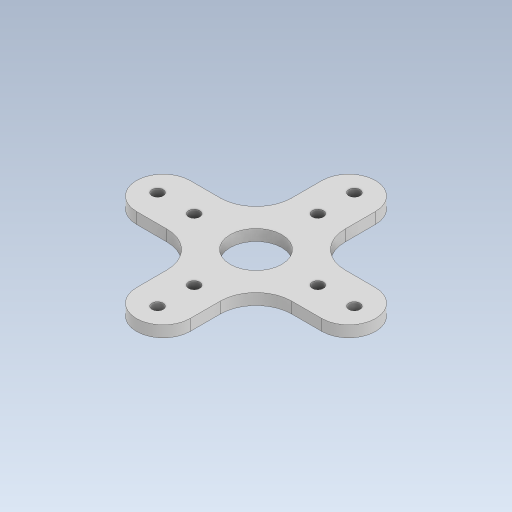
# Autodesk Inventor part: DriveMotorPlate
Saved by Autodesk Inventor 2023 (Build 270158000, 158)
## iProperties
Created: 2023-03-28
Part Number: DriveMotorPlate
Material: Generic
Document SubType Name: Modeling
Designer: Dave
Density: 1 g/cm^3
Appearance: Default
Author: Dave
Autodesk Inventor part; units mm, degrees
ref_plane "YZ Plane" through (0, 0, 0) normal (1, 0, 0) x (0, 1, 0)
ref_plane "XZ Plane" through (0, 0, 0) normal (0, 1, 0) x (-1, 0, 0)
ref_plane "XY Plane" through (0, 0, 0) normal (0, 0, 1) x (1, 0, 0)
sketch "Sketch1" plane through (0, 0, 0) normal (0, 1, 0) x (-1, 0, 0)
  line L0 (-9.525, -33) -> (-9.525, -22.225)
  line L1 (-9.525, 22.225) -> (-9.525, 33)
  line L2 (33, 9.525) -> (22.225, 9.525)
  line L3 (-22.225, 9.525) -> (-33, 9.525)
  line L4 (9.525, 33) -> (9.525, 22.225)
  line L5 (9.525, -22.225) -> (9.525, -33)
  line L6 (-33, -9.525) -> (-22.225, -9.525)
  line L7 (22.225, -9.525) -> (33, -9.525)
  line L8 (77.6073, 0) -> (-79.7857, 0) projected
  line L9 (0, -77.9019) -> (0, 71.2895) projected
  circle A0 centre (-35, 0) radius 2
  circle A1 centre (-22, 0) radius 2
  circle A2 centre (0, -22) radius 2
  circle A3 centre (0, -35) radius 2
  circle A4 centre (22, 0) radius 2
  circle A5 centre (35, 0) radius 2
  circle A6 centre (0, 22) radius 2
  circle A7 centre (0, 35) radius 2
  circle A8 centre (0, 0) radius 9.185
  line L10 (-57.3009, 49.9764) -> (55.1226, 49.9764) construction
  line L11 (55.1226, 49.9764) -> (55.1226, -56.5889) construction
  line L12 (55.1226, -56.5889) -> (-57.3009, -56.5889) construction
  line L13 (-57.3009, -56.5889) -> (-57.3009, 49.9764) construction
  arc A9 (9.525, 33) -> (0, 42.525) centre (0, 33) ccw
  arc A10 (0, 42.525) -> (-9.525, 33) centre (0, 33) ccw
  arc A11 (42.525, 0) -> (33, 9.525) centre (33, 0) ccw
  arc A12 (33, -9.525) -> (42.525, 0) centre (33, 0) ccw
  arc A13 (0, -42.525) -> (9.525, -33) centre (0, -33) ccw
  arc A14 (-9.525, -33) -> (0, -42.525) centre (0, -33) ccw
  arc A15 (-42.525, 0) -> (-33, -9.525) centre (-33, 0) ccw
  arc A16 (-33, 9.525) -> (-42.525, 0) centre (-33, 0) ccw
  arc A17 (9.525, 22.225) -> (22.225, 9.525) centre (22.225, 22.225) ccw
  arc A18 (22.225, -9.525) -> (9.525, -22.225) centre (22.225, -22.225) ccw
  arc A19 (-9.525, -22.225) -> (-22.225, -9.525) centre (-22.225, -22.225) ccw
  arc A20 (-22.225, 9.525) -> (-9.525, 22.225) centre (-22.225, 22.225) ccw
  point P0 (0, 42.525)
  point P1 (42.525, 0)
  point P2 (0, -42.525)
  point P3 (-42.525, 0)
  point P4 (42.525, 0)
  point P5 (0, 42.525)
  point P6 (-42.525, 0)
  dimension "d2" = 360
  dimension "d4" = 4
  dimension "d5" = 22
  dimension "d6" = 35
  dimension "d7" = 18.37
  dimension "d39" = 9.525
  dimension "d41" = 9.525
  dimension "d46" = 12.7
  constraints: 24 point on circle, 20 centre point, 16 end point, 16 tangent, 10 equal radius, 8 parallel, 7 point on line, 4 horizontal, 3 perpendicular, 3 vertical, 1 coincident, 1 vertical alignment, 45 other
  measures "d4" diameter of A0
  measures "d5" distance from line of A1.centre L9
  measures "d6" distance from line of L9 A0.centre
  measures "d7" diameter of A8
  measures "d39" radius of A9
  measures "d41" radius of A14
  measures "d46" radius of A17
extrude "Extrusion1" add sketch "Sketch1" along normal blind 4 contours L0 A19 L6 A15 L8 A0 A1 A8 L9 A2 A3 A14 | L9 A3 A2 A8 L8 A4 A5 A12 L7 A18 L5 A13 | A16 L3 A20 L1 A10 L9 A7 A6 A8 L8 A1 A0 | L8 A5 A4 A8 L9 A6 A7 A9 L4 A17 L2 A11
body "Solid1"
